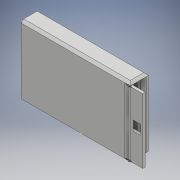
# Autodesk Inventor part: CardBox_4slots_B
Saved by Autodesk Inventor 2018 (Build 220112000, 112)
## iProperties
Created: 2019-03-10
Part Number: CardBox_4slots_B
Material: Generic
Document SubType Name: Modeling
Designer: natha
Density: 1 g/cm^3
Appearance: Default
Author: natha
Autodesk Inventor part; units mm, degrees
ref_plane "YZ Plane" through (0, 0, 0) normal (1, 0, 0) x (0, 1, 0)
ref_plane "XZ Plane" through (0, 0, 0) normal (0, 1, 0) x (-1, 0, 0)
ref_plane "XY Plane" through (0, 0, 0) normal (0, 0, 1) x (1, 0, 0)
sketch "Sketch1" plane through (0, 0, 0) normal (0, 0, 1) x (1, 0, 0)
  line L0 (-51.9238, 7.67) -> (40.5487, 7.67)
  line L1 (50.9762, -5.53) -> (50.9762, -7.53)
  line L2 (50.9762, -7.53) -> (-51.9238, -7.53)
  line L3 (-51.9238, -7.53) -> (-51.9238, 7.67)
  line L4 (-51.9238, 7.67) -> (50.9762, -7.53) construction
  line L5 (50.8142, 7.3691) -> (-51.9238, -7.53) construction
  line L6 (40.55, -5.53) -> (50.9762, -5.53)
  line L7 (40.5487, 5.67) -> (-49.9238, 5.67)
  line L8 (-49.9238, 5.67) -> (-49.9238, 3.42)
  line L9 (-49.9238, 3.42) -> (38.3707, 3.42)
  line L10 (40.5487, 7.67) -> (40.5487, 5.8804)
  line L11 (40.55, -5.53) -> (-49.9238, -5.53)
  line L12 (-49.9238, -5.53) -> (-49.9238, -3.28)
  line L13 (-49.9238, -3.28) -> (38.3707, -3.28)
  line L14 (40.5487, 5.8804) -> (40.5487, 5.67)
  line L15 (38.3707, 2.82) -> (-49.9238, 2.82)
  line L16 (-49.9238, 2.82) -> (-49.9238, 0.57)
  line L17 (-49.9238, 0.57) -> (38.3707, 0.57)
  line L18 (38.3707, 3.42) -> (38.3707, 2.82)
  line L19 (38.3707, -0.03) -> (-49.9238, -0.03)
  line L20 (-49.9238, -0.03) -> (-49.9238, -2.28)
  line L21 (-49.9238, -2.28) -> (38.3707, -2.28)
  line L22 (38.3707, 0.57) -> (38.3707, -0.03)
  line L23 (38.3707, -2.28) -> (38.3707, -3.28)
  point P0 (0, 0)
  dimension "d0" = 102.9
  dimension "d1" = 14.9
  dimension "d3" = 2
  dimension "d4" = 2
  dimension "d5" = 2.25
  dimension "d6" = 2
  dimension "d7" = 2
  dimension "d8" = 2.25
  dimension "d10" = 0.6
  dimension "d11" = 2.25
  dimension "d12" = 2
  dimension "d13" = 0.6
  dimension "d14" = 2.25
  dimension "d15" = 1
  dimension "d16" = 2
  constraints: 48 end point, 15 perpendicular, 4 horizontal, 4 point on line, 3 parallel, 2 vertical
  measures "d0" distance of L1.end L2.end
  measures "d1" distance of L5.start L1.end
  measures "d3" distance between parallel lines of L2 L6
  measures "d4" distance between parallel lines of L7 L0
  measures "d5" distance between parallel lines of L9 L7
  measures "d6" distance between parallel lines of L3 L8
  measures "d7" distance between parallel lines of L3 L12
  measures "d8" distance between parallel lines of L11 L13
  measures "d10" distance between parallel lines of L15 L9
  measures "d11" distance between parallel lines of L17 L15
  measures "d12" distance between parallel lines of L3 L16
  measures "d13" distance between parallel lines of L19 L17
  measures "d14" distance between parallel lines of L21 L19
  measures "d15" distance between parallel lines of L13 L21
  measures "d16" distance between parallel lines of L3 L20
extrude "Extrusion1" add sketch "Sketch1" along normal blind 54.5
sketch "Sketch2" plane through (0, 0, 54.5) normal (0, 0, 1) x (1, 0, 0)
  line L0 (-51.9238, 7.67) -> (40.5487, 7.67) projected
  line L1 (50.9762, -7.53) -> (-51.9238, -7.53) projected
  line L2 (40.5487, 7.67) -> (-51.9238, 7.67)
  line L3 (-51.9238, 7.67) -> (-51.9238, -7.53)
  line L4 (-51.9238, -7.53) -> (40.5487, -7.53)
  line L5 (40.5487, -7.53) -> (40.5487, 7.67)
  point P0 (0, 0)
  constraints: 8 end point, 2 parallel, 1 horizontal, 1 perpendicular
extrude "Extrusion2" add sketch "Sketch2" along normal blind 2
sketch "Sketch3" plane through (0, 0, 0) normal (0, 0, -1) x (-1, 0, 0)
  line L0 (-40.5487, 7.67) -> (-40.5487, 5.67) projected
  line L1 (51.9238, -7.53) -> (51.9238, 7.67) projected
  line L2 (-40.5487, 7.67) -> (51.9238, 7.67)
  line L3 (51.9238, 7.67) -> (51.9238, -7.53)
  line L4 (51.9238, -7.53) -> (-40.5487, -7.53)
  line L5 (-40.5487, -7.53) -> (-40.5487, 7.67)
  point P0 (0, 0)
  constraints: 8 end point, 2 parallel, 1 horizontal, 1 perpendicular
extrude "Extrusion3" add sketch "Sketch3" along normal blind 2
sketch "Sketch4" plane through (40.5487, -7.53, 0) normal (0, -1, 0) x (1, 0, 0)
  line L0 (8.4275, 31.25) -> (2.4275, 31.25)
  line L1 (2.4275, 31.25) -> (2.4275, 23.25)
  line L2 (2.4275, 23.25) -> (8.4275, 23.25)
  line L3 (8.4275, 23.25) -> (8.4275, 31.25)
  line L4 (10.4275, 0) -> (10.4275, 54.5) projected
  line L5 (10.4275, 0) -> (0, 0) projected
  point P0 (-40.5487, 0)
  dimension "d23" = 2
  dimension "d24" = 8
  dimension "d25" = 6
  dimension "d26" = 23.25
  constraints: 8 end point, 2 parallel, 1 horizontal, 1 perpendicular
  measures "d23" distance between parallel lines of L4 L3
  measures "d24" distance between parallel lines of L2 L0
  measures "d25" distance between parallel lines of L3 L1
  measures "d26" distance between parallel lines of L5 L2
extrude "Extrusion4" cut sketch "Sketch4" against normal blind 2
chamfer "Chamfer1" distance 2 angle 45 10 edges at (-5.6875, 7.67, -2) (-5.6875, -7.53, -2) (-51.9238, 0.07, -2) (-51.9238, 7.67, 27.25) (-5.6875, 7.67, 56.5) (-51.9238, -7.53, 27.25) (-5.6875, -7.53, 56.5) (-51.9238, 0.07, 56.5) (40.5487, 0.07, -2) (40.5487, 0.07, 56.5)
sketch "Sketch5" plane through (50.9762, -7.53, 0) normal (0, -1, 0) x (1, 0, 0)
  point P0 (-50.9762, 0)
sketch "Sketch6" plane through (50.9762, -7.53, 0) normal (0, -1, 0) x (1, 0, 0)
  line L0 (-12.6056, 0) -> (-12.6056, 54.5) projected
  line L1 (-12.6056, 54) -> (-13.1056, 54)
  line L2 (-13.1056, 54) -> (-13.1056, 0.5)
  line L3 (-13.1056, 0.5) -> (-12.6056, 0.5)
  line L4 (-12.6056, 0.5) -> (-12.6056, 54)
  line L5 (-100.9, 54.5) -> (-10.4275, 54.5) projected
  line L6 (-10.4275, 0) -> (-100.9, 0) projected
  point P0 (-50.9762, 0)
  dimension "d32" = 0.5
  dimension "d33" = 0.5
  dimension "d34" = 0.5
  constraints: 8 end point, 2 parallel, 1 horizontal, 1 perpendicular, 1 point on line
  measures "d32" distance between parallel lines of L5 L1
  measures "d33" distance between parallel lines of L0 L2
  measures "d34" distance between parallel lines of L6 L3
extrude "Extrusion5" cut sketch "Sketch6" against normal blind 2
fillet "Fillet1" radius 2 2 edges at (38.3707, -7.53, 27.25) (37.8707, -7.53, 27.25)
sketch "Sketch7" plane through (50.9762, -7.53, 0) normal (0, -1, 0) x (1, 0, 0)
  line L0 (-100.9, 0) -> (-10.4275, 0) projected
  line L1 (0, 0) -> (0, 54.5) projected
  line L2 (-10.4275, 0) -> (0, 0)
  line L3 (0, 0) -> (0, 0.3)
  line L4 (0, 0.3) -> (-10.4275, 0.3)
  line L5 (-10.4275, 0.3) -> (-10.4275, 0)
  point P0 (-50.9762, 0)
  dimension "d38" = 0.3
  constraints: 8 end point, 2 parallel, 1 horizontal, 1 perpendicular, 1 point on line
  measures "d38" distance between parallel lines of L2 L4
extrude "Extrusion6" cut sketch "Sketch7" against normal blind 2
sketch "Sketch8" plane through (-49.9238, -7.53, 54.5) normal (0, -1, 0) x (1, 0, 0)
  line L0 (100.9, -54.2) -> (100.9, 0) projected
  line L1 (100.9, 0) -> (90.3928, 0)
  line L2 (90.3928, 0) -> (90.3928, -0.3)
  line L3 (90.3928, -0.3) -> (100.9, -0.3)
  line L4 (100.9, -0.3) -> (100.9, 0)
  point P0 (49.9238, -54.5)
  dimension "d41" = 0.3
  constraints: 8 end point, 2 parallel, 1 horizontal, 1 perpendicular
  measures "d41" distance between parallel lines of L1 L3
extrude "Extrusion7" cut sketch "Sketch8" against normal blind 2
sketch "Sketch9" plane through (-49.9238, -7.53, 0) normal (0, -1, 0) x (1, 0, 0)
  line L0 (88.2944, 0) -> (88.2944, 54.5) projected
  line L1 (88.2944, 54) -> (90.2944, 54) projected
  line L2 (88.2944, 54.2) -> (88.6944, 54.2)
  line L3 (88.6944, 54.2) -> (88.6944, 54)
  line L4 (88.6944, 54) -> (88.2944, 54)
  line L5 (88.2944, 54) -> (88.2944, 54.2)
  line L6 (88.2944, 0) -> (88.2944, 54.5) projected
  line L7 (88.2944, 0.4862) -> (88.6944, 0.4862)
  line L8 (88.6944, 0.4862) -> (88.6944, 0.2862)
  line L9 (88.6944, 0.2862) -> (88.2944, 0.2862)
  line L10 (88.2944, 0.2862) -> (88.2944, 0.4862)
  point P0 (49.9238, 0)
  dimension "d44" = 0.2
  dimension "d45" = 0.4
  dimension "d46" = 0.2
  dimension "d47" = 0.4
  constraints: 16 end point, 4 parallel, 3 point on line, 2 horizontal, 2 perpendicular
  measures "d44" distance between parallel lines of L1 L2
  measures "d45" distance between parallel lines of L3 L0
  measures "d46" distance between parallel lines of L9 L7
  measures "d47" distance between parallel lines of L8 L0
extrude "Extrusion8" cut sketch "Sketch9" against normal blind 2
sketch "Sketch10" plane through (-49.9238, -7.53, 0) normal (0, -1, 0) x (1, 0, 0)
  line L0 (90.2944, 0.5) -> (88.2944, 0.5) projected
  line L1 (88.2944, 0.5) -> (88.6944, 0.5)
  line L2 (88.6944, 0.5) -> (88.6944, 0.4862)
  line L3 (88.6944, 0.4862) -> (88.2944, 0.4862)
  line L4 (88.2944, 0.4862) -> (88.2944, 0.5)
  point P0 (49.9238, 0)
  constraints: 8 end point, 2 parallel, 1 horizontal, 1 perpendicular
extrude "Extrusion9" cut sketch "Sketch10" against normal blind 2
sketch "Sketch11" plane through (-49.9238, -7.53, 0) normal (0, -1, 0) x (1, 0, 0)
  line L0 (90.3928, 54.2) -> (90.3928, 54.5) projected
  line L1 (88.6944, 54) -> (90.2944, 54) projected
  line L2 (90.3928, 54.2) -> (89.6944, 54.2)
  line L3 (89.6944, 54.2) -> (89.6944, 54)
  line L4 (89.6944, 54) -> (90.3928, 54)
  line L5 (90.3928, 54) -> (90.3928, 54.2)
  line L6 (88.6944, 54.2) -> (88.6944, 54) projected
  line L7 (90.4725, 0.3) -> (90.4725, 0) projected
  line L8 (90.2944, 0.5) -> (88.6944, 0.5) projected
  line L9 (90.4725, 0.3) -> (89.6944, 0.3)
  line L10 (89.6944, 0.3) -> (89.6944, 0.5)
  line L11 (89.6944, 0.5) -> (90.4725, 0.5)
  line L12 (90.4725, 0.5) -> (90.4725, 0.3)
  line L13 (88.6944, 0.5) -> (88.6944, 0.2862) projected
  point P0 (49.9238, 0)
  dimension "d52" = 1
  dimension "d53" = 1
  constraints: 16 end point, 4 parallel, 2 horizontal, 2 perpendicular, 2 point on line
  measures "d52" distance between parallel lines of L3 L6
  measures "d53" distance between parallel lines of L10 L13
chamfer "Chamfer2" distance 2 angle 45 2 edges at (42.9762, -5.53, 27.25) (48.9762, -5.53, 27.25)
body "Solid1"
